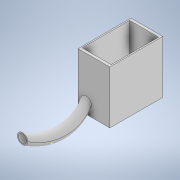
# Autodesk Inventor part: sugar
Saved by Autodesk Inventor 2021 (Build 250183000, 183)
## iProperties
Created: 2020-10-16
Part Number: sugar
Material: Generic
Document SubType Name: Modeling
Designer: David
Density: 1 g/cm^3
Appearance: Default
Author: David
Autodesk Inventor part; units mm, degrees
ref_plane "YZ Plane" through (0, 0, 0) normal (1, 0, 0) x (0, 1, 0)
ref_plane "XZ Plane" through (0, 0, 0) normal (0, 1, 0) x (-1, 0, 0)
ref_plane "XY Plane" through (0, 0, 0) normal (0, 0, 1) x (1, 0, 0)
sketch "Sketch1" plane through (0, 0, 0) normal (0, 1, 0) x (-1, 0, 0)
  line L0 (38.1, -63.5) -> (-38.1, -63.5)
  line L1 (-38.1, -63.5) -> (-38.1, 63.5)
  line L2 (-38.1, 63.5) -> (38.1, 63.5)
  line L3 (38.1, 63.5) -> (38.1, -63.5)
  point P0 (0, 0)
  point P1 (38.1, 0)
  dimension "d0" = 76.2
  dimension "d1" = 127
  dimension "d2" = 38.1
  constraints: 8 end point, 2 parallel, 1 horizontal, 1 horizontal alignment, 1 midpoint, 1 perpendicular
  measures "d0" distance of L1.end L2.end
  measures "d1" distance of L2.end L0.start
  measures "d2" distance from line of L3 point (0, 0)
extrude "Extrusion1" add sketch "Sketch1" along normal blind 38.1
sketch "Sketch2" plane through (0, 38.1, 0) normal (0, 1, 0) x (1, 0, 0)
  line L0 (-38.1, 63.5) -> (-38.1, -63.5) projected
  line L1 (-38.1, -63.5) -> (38.1, -63.5) projected
  line L2 (-38.1, 63.5) -> (38.1, 63.5)
  line L3 (38.1, 63.5) -> (38.1, -63.5)
  line L4 (38.1, -63.5) -> (-38.1, -63.5)
  line L5 (-38.1, -63.5) -> (-38.1, 63.5)
  line L6 (-34.925, 57.15) -> (34.925, 57.15)
  line L7 (34.925, 57.15) -> (34.925, -57.15)
  line L8 (34.925, -57.15) -> (-34.925, -57.15)
  line L9 (-34.925, -57.15) -> (-34.925, 57.15)
  point P0 (0, 0)
  point P1 (-34.925, 0)
  point P2 (0, -57.15)
  point P3 (0, -63.5)
  dimension "d5" = 114.3
  dimension "d6" = 69.85
  constraints: 16 end point, 4 parallel, 3 midpoint, 2 horizontal, 2 perpendicular, 1 horizontal alignment, 1 vertical alignment
  measures "d5" distance of L8.end L6.start
  measures "d6" distance of L7.end L8.end
extrude "Extrusion2" add sketch "Sketch2" along normal blind 88.9
sketch "Sketch3" plane through (-38.1, 0, 63.5) normal (0, 0, 1) x (1, 0, 0)
  circle A0 centre (19.05, 25.4) radius 12.7
  line L0 (0, 0) -> (76.2, 0) projected
  line L1 (0, 0) -> (0, 127) projected
  circle A1 centre (19.05, 25.4) radius 10.16
  point P0 (38.1, 0)
  dimension "d9" = 25.4
  dimension "d10" = 25.4
  dimension "d11" = 19.05
  dimension "d17" = 20.32
  constraints: 2 centre point, 1 coincident
  measures "d9" diameter of A0
  measures "d10" distance from line of A0.centre L0
  measures "d11" distance from line of A0.centre L1
  measures "d17" diameter of A1
ref_plane "Work Plane1" through (-38.1, 0, 165.1) normal (0, 0, 1) x (1, 0, 0)
sketch "Sketch4" plane through (-38.1, 0, 165.1) normal (0, 0, 1) x (1, 0, 0)
  circle A0 centre (-31.75, -25.4) radius 12.7
  line L0 (0, 0) -> (76.2, 0) projected
  line L1 (0, 0) -> (0, 127) projected
  line L2 (76.2, 0) -> (76.2, 127) projected
  circle A1 centre (19.05, 25.4) radius 12.7 projected
  circle A2 centre (-31.75, -25.4) radius 10.16
  point P0 (38.1, 0)
  dimension "d13" = 50.8
  dimension "d14" = 25.4
  dimension "d18" = 20.32
  constraints: 2 centre point, 1 coincident, 1 equal radius
  measures "d13" horizontal distance of A0.centre A1.centre
  measures "d14" distance from line of L0 A0.centre
  measures "d18" diameter of A2
sketch3d "3D Sketch1"
  arc A0 (-69.85, -25.4, 165.1) -> (-19.05, 25.4, 63.5) centre (-76.6593, 57.7635, 127.0771) ccw
  dimension "d19" = 101.6
sweep "Sweep1" add profiles "Sketch4" path "3D Sketch1" keep normal constant yes contours A0
extrude "Extrusion3" cut sketch "Sketch3" against normal blind 25.4 contours A1
sketch "Sketch12" plane through (-34.925, 38.1, -57.15) normal (0, 0, 1) x (1, 0, 0)
  line L0 (0, 0) -> (0, 88.9) projected
  line L1 (0, 31.5422) -> (69.85, 31.5422)
  line L2 (69.85, 31.5422) -> (69.85, 0)
  line L3 (69.85, 0) -> (0, 0)
  line L4 (0, 0) -> (0, 31.5422)
  line L5 (69.85, 0) -> (69.85, 88.9) projected
  point P0 (34.925, -38.1)
  constraints: 8 end point, 2 parallel, 1 collinear, 1 horizontal, 1 perpendicular, 1 point on line
loft "Loft1" cut profiles "Sketch12" section 2 edges at (-31.75, 25.4, 63.5)
sketch "Sketch13" plane through (-38.1, 0, 165.1) normal (0, 0, 1) x (1, 0, 0)
  point P0 (38.1, 0)
body "Solid1"
